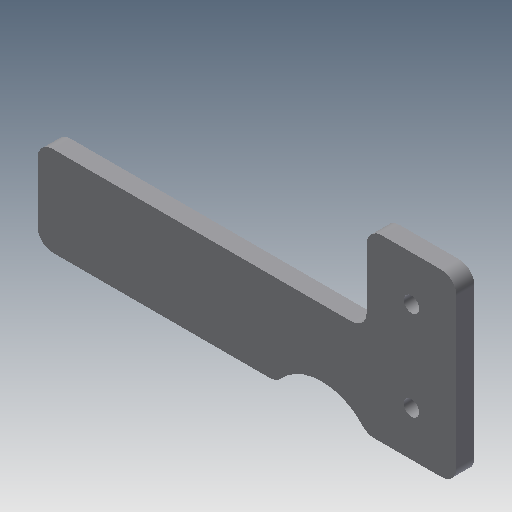
# Autodesk Inventor part: Spool Holder
Saved by Autodesk Inventor 2017 (Build 210142000, 142)
## iProperties
Created: 2016-06-13
Part Number: Spool Holder
Material: Generic
Document SubType Name: Modeling
Designer: joshmamo
Density: 1 g/cm^3
Appearance: Default
Author: joshmamo
Autodesk Inventor part; units mm, degrees
ref_plane "YZ Plane" through (0, 0, 0) normal (1, 0, 0) x (0, 1, 0)
ref_plane "XZ Plane" through (0, 0, 0) normal (0, 1, 0) x (-1, 0, 0)
ref_plane "XY Plane" through (0, 0, 0) normal (0, 0, 1) x (1, 0, 0)
sketch "Sketch1" plane through (0, 0, 0) normal (0, 0, 1) x (1, 0, 0)
  line L0 (5.4828, 0) -> (-17.1232, 0)
  line L1 (-129.5172, 5) -> (-129.5172, 25)
  line L2 (-14.5018, 60) -> (5.4828, 60)
  line L3 (10.4828, 55) -> (10.4828, 5)
  arc A0 (-20.8273, 1.6415) -> (-48.1762, 1.6415) centre (-34.5018, -10.7569) ccw
  line L4 (-129.5172, 5) -> (-129.5172, 25)
  line L5 (-124.5172, 30) -> (-24.5018, 30)
  line L6 (-19.5018, 35) -> (-19.5018, 55)
  arc A1 (-24.5018, 30) -> (-19.5018, 35) centre (-24.5018, 35) ccw
  arc A2 (10.4828, 55) -> (5.4828, 60) centre (5.4828, 55) ccw
  arc A3 (5.4828, 0) -> (10.4828, 5) centre (5.4828, 5) ccw
  arc A4 (-129.5172, 5) -> (-124.5172, 0) centre (-124.5172, 5) ccw
  arc A5 (-124.5172, 30) -> (-129.5172, 25) centre (-124.5172, 25) ccw
  arc A6 (-14.5018, 60) -> (-19.5018, 55) centre (-14.5018, 55) ccw
  arc A7 (-20.8273, 1.6415) -> (-17.1232, 0) centre (-17.1232, 5) ccw
  line L7 (-51.8804, 0) -> (-124.5172, 0)
  arc A8 (-51.8804, 0) -> (-48.1762, 1.6415) centre (-51.8804, 5) ccw
  line L8 (-4.5095, 60) -> (-4.5429, 0) construction
  line L9 (-4.5429, 0) -> (10.4571, 0) construction
  circle A9 centre (-4.5429, 15) radius 2.6
  circle A10 centre (-4.5178, 45) radius 2.6
  point P0 (0, 0)
  point P1 (10.4828, 60)
  point P2 (-129.5172, 30)
  dimension "d5" = 5
  dimension "d6" = 5
  dimension "d8" = 5
  dimension "d9" = 5
  dimension "d10" = 5
  dimension "d11" = 5
  dimension "d12" = 5
  dimension "d14" = 60
  dimension "d18" = 5.2
  dimension "d19" = 5.2
  constraints: 20 end point, 18 point on circle, 14 tangent, 11 centre point, 7 point on line, 3 horizontal, 3 perpendicular, 2 parallel, 1 midpoint
  measures "d5" radius of A2
  measures "d6" radius of A3
  measures "d8" radius of A4
  measures "d9" radius of A5
  measures "d10" radius of A6
  measures "d11" radius of A7
  measures "d12" radius of A8
  measures "d14" distance of L8.start L8.end
  measures "d18" diameter of A9
  measures "d19" diameter of A10
extrude "Extrusion1" add sketch "Sketch1" along normal blind 6
body "Solid1"
